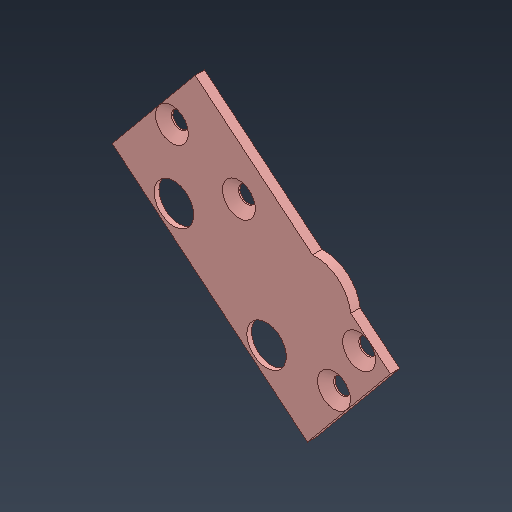
# Autodesk Inventor part: gearbox-holder-wall-left
Saved by Autodesk Inventor 2023 (Build 270158000, 158)
## iProperties
Created: 2025-04-06
Part Number: gearbox-holder-wall-left
Material: ABS Plastic
Document SubType Name: Modeling
Designer: szymo
Density: 1.06 g/cm^3
Appearance: Default(1)
Mass: 2.61994 g
Surface Area: 32.3954 cm^2
Volume: 2.47164 cm^3
Author: szymo
Autodesk Inventor part; units mm, degrees
ref_plane "YZ Plane" through (0, 0, 0) normal (1, 0, 0) x (0, 1, 0)
ref_plane "XZ Plane" through (0, 0, 0) normal (0, 1, 0) x (-1, 0, 0)
ref_plane "XY Plane" through (0, 0, 0) normal (0, 0, 1) x (1, 0, 0)
ref_plane "Work Plane1" through (29.5652, -6.4288, 0) normal (0, 0, 1) x (0.7715113, -0.6362157, 0)
ref_plane "Work Plane5" through (29.5652, -6.4288, 0.1) normal (0, 0, 1) x (0.7715113, -0.6362157, 0)
sketch "Sketch2" plane through (29.5652, -6.4288, 0.1) normal (0, 0, 1) x (0.7715113, -0.6362157, 0)
  line L0 (-5.5466, -27.7) -> (0, -27.7) projected
  line L1 (0, -27.7) -> (0, 0) projected
  line L2 (0, 0) -> (-10.933, 0) projected
  arc A0 (-10.933, 0) -> (-21.4476, 0) centre (-16.1903, -5.4188) ccw projected
  line L3 (-21.4476, 0) -> (-53.8, 0) projected
  line L4 (-53.8, 0) -> (-53.8, -27.7) projected
  line L5 (-53.8, -27.7) -> (-50.5534, -27.7) projected
  arc A1 (-31.0466, -27.7) -> (-50.5534, -27.7) centre (-40.8, -22.8337) ccw projected
  line L6 (-31.0466, -27.7) -> (-25.0534, -27.7) projected
  arc A2 (-5.5466, -27.7) -> (-25.0534, -27.7) centre (-15.3, -22.8337) ccw projected
  circle A3 centre (-40.8, -22.8337) radius 6 projected
  circle A4 centre (-15.3, -22.8337) radius 6 projected
  circle A5 centre (-40.8, -22.8337) radius 6.2
  circle A6 centre (-15.3, -22.8337) radius 6.2
  line L7 (-50.5534, -27.7) -> (-5.5466, -27.7)
  point P0 (-26.9, -13.85)
  point P1 (-44.6418, -27.7)
  point P2 (-36.9582, -27.7)
  point P3 (-19.1418, -27.7)
  point P4 (-11.4582, -27.7)
  dimension "d2" = 0.2
  dimension "d3" = 0.2
  constraints: 2 centre point, 2 end point, 1 horizontal
  measures "d2" radial gap between concentric circles of A3 A5
  measures "d3" radial gap between concentric circles of A4 A6
ref_plane "Work Plane2" through (-24.886, -6.534, 1.1) normal (0, 0, 1) x (0.7715113, -0.6362157, 0)
extrude "Extrusion2" add sketch "Sketch2" along normal up to surface (1 mm away) contours A2 L6 A1 L5 L4 L3 A0 L2 L1 L0 | L7 A6 A2 | L7 A5 A1
ref_plane "Work Plane6" through (-11.9421, 27.7996, 1.1) normal (0, 0, 1) x (0.7715113, -0.6362157, 0)
sketch "Sketch3" plane through (-11.9421, 27.7996, 1.1) normal (0, 0, 1) x (0.7715113, -0.6362157, 0)
  line L0 (0, -27.7) -> (0, 0) projected
  line L1 (9.1582, -27.7) -> (0, -27.7) projected
  arc A0 (16.8418, -27.7) -> (9.1582, -27.7) centre (13, -22.8337) ccw projected
  line L2 (34.6582, -27.7) -> (16.8418, -27.7) projected
  arc A1 (42.3418, -27.7) -> (34.6582, -27.7) centre (38.5, -22.8337) ccw projected
  line L3 (53.8, -27.7) -> (42.3418, -27.7) projected
  line L4 (53.8, 0) -> (53.8, -27.7) projected
  line L5 (42.867, 0) -> (53.8, 0) projected
  line L6 (0, 0) -> (32.3524, 0) projected
  circle A2 centre (13, -22.8337) radius 4 projected
  circle A3 centre (38.5, -22.8337) radius 4 projected
  circle A4 centre (13, -22.8337) radius 4.2
  circle A5 centre (38.5, -22.8337) radius 4.2
  line L7 (9.1582, -27.7) -> (42.3418, -27.7)
  arc A6 (42.867, 0) -> (32.3524, 0) centre (37.6097, -5.4188) ccw projected
  point P0 (26.9, -13.85)
  point P1 (16.8418, -27.7)
  point P2 (34.6582, -27.7)
  point P3 (16.8418, -27.7)
  point P4 (34.6582, -27.7)
  dimension "d6" = 0.2
  dimension "d7" = 0.2
  constraints: 2 centre point, 2 end point, 1 horizontal
  measures "d6" radial gap between concentric circles of A2 A4
  measures "d7" radial gap between concentric circles of A3 A5
ref_plane "Work Plane3" through (-22.0705, -3.7186, 2.1) normal (0, 0, 1) x (0.7715113, -0.6362157, 0)
extrude "Extrusion3" add sketch "Sketch3" along normal up to surface (1 mm away) contours L0 L6 A6 L5 L4 L3 A1 L2 A0 L1 | A0 L7 | A1 L7
ref_plane "Work Plane4" through (29.5652, -6.4288, 0) normal (0, 0, -1) x (-0.7715113, 0.6362157, 0)
sketch "Sketch4" plane through (29.5652, -6.4288, 0) normal (0, 0, -1) x (-0.7715113, 0.6362157, 0)
  circle A0 centre (28.05, -17.6859) radius 1.25 projected
  circle A1 centre (24.4296, -8.3643) radius 1.25 projected
  circle A2 centre (16.1903, -5.4188) radius 1.25 projected
  circle A3 centre (24.4296, -8.3643) radius 1.55
  circle A4 centre (28.05, -17.6859) radius 1.55
  circle A5 centre (16.1903, -5.4188) radius 1.55
  point P0 (26.9, -13.85)
  dimension "d10" = 0.3
  dimension "d11" = 0.3
  dimension "d12" = 0.3
  constraints: 3 centre point
  measures "d10" radial gap between concentric circles of A1 A3
  measures "d11" radial gap between concentric circles of A0 A4
  measures "d12" radial gap between concentric circles of A2 A5
extrude "Extrusion4" cut sketch "Sketch4" against normal blind 1.6 contours A0 | A1 | A2 | A3 | A4 | A5
sketch "Sketch5" plane through (-29.5652, 6.4288, 2.1) normal (0, 0, 1) x (0.7715113, -0.6362157, 0)
  circle A0 centre (50.3, 13.1197) radius 2.5 projected
  circle A1 centre (18.7242, 19.6186) radius 2.5 projected
  circle A2 centre (3.5, 15.688) radius 2.5 projected
  line L0 (0, 0) -> (3.2466, 0) projected
  arc A3 (18.5089, 14.2717) -> (3.2466, 0) centre (13, 4.8663) ccw projected
  arc A4 (22.4055, 17.7195) -> (18.5089, 14.2717) centre (25.75, 10.0141) ccw projected
  arc A5 (31.5863, 26.1337) -> (22.4055, 17.7195) centre (29.3704, 19.3357) ccw projected
  arc A6 (43.3624, 18.0351) -> (31.5863, 26.1337) centre (37.6097, 22.2812) ccw projected
  arc A7 (45.328, 13.3627) -> (43.3624, 18.0351) centre (39.95, 13.85) ccw projected
  arc A8 (48.2534, 0) -> (45.328, 13.3627) centre (38.5, 4.8663) ccw projected
  line L1 (48.2534, 0) -> (53.8, 0) projected
  line L2 (53.8, 0) -> (53.8, 27.7) projected
  line L3 (53.8, 27.7) -> (42.867, 27.7) projected
  arc A9 (42.867, 27.7) -> (32.3524, 27.7) centre (37.6097, 22.2812) ccw projected
  line L4 (32.3524, 27.7) -> (0, 27.7) projected
  line L5 (0, 27.7) -> (0, 0) projected
  circle A10 centre (48.0855, 24.2) radius 2.5 projected
  point P0 (26.9, 13.85)
  constraints: 3 coincident
hole "Hole1" at (-16.884, 16.3055, 2.1) at (-2.6376, 9.6522, 2.1) at (17.5888, -15.4508, 2.1) at (22.9296, -5.4934, 2.1) direction (0, 0, -1) diameter 3.6 end through all countersink diameter 7 countersink angle 90 clearance for "Countersunk Flat Head Screw ISO 2009/7046" size "M3" standard "ISO"
body "Solid1"
